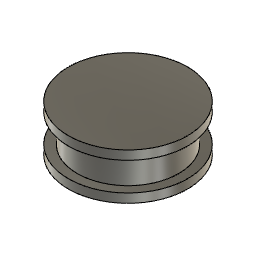
LaufradVorlage (Autodesk Fusion 360 design; units mm, degrees)
Autodesk Fusion 360 part; units mm, degrees
sketch "Skizze1" plane through (0, 0, 0) normal (0, 0, 1) x (1, 0, 0)
  circle A0 centre (0, 0) radius 17
  dimension "d1" = 34
  constraint coincident A0.centre origin
  measures "d1" diameter of A0
extrude "Extrusion1" add sketch "Skizze1" along normal blind 9.5
sketch "Skizze2" plane through (0, 0, 9.5) normal (0, 0, 1) x (-1, 0, 0)
  circle A0 centre (0, 0) radius 17
  circle A1 centre (0, 0) radius 20
  dimension "d5" = 40
  constraint coincident A0.centre A1.centre
  measures "d5" diameter of A1
extrude "Extrusion2" add sketch "Skizze2" along normal blind 3 contours A0 | A1
sketch "Skizze3" plane through (0, 0, 0) normal (0, 0, -1) x (1, 0, 0)
  circle A0 centre (0, 0) radius 17
  circle A1 centre (0, 0) radius 20
  dimension "d8" = 40
  constraint coincident A0.centre A1.centre
  measures "d8" diameter of A1
extrude "Extrusion3" add sketch "Skizze3" along normal blind 3 contours A0 | A1
